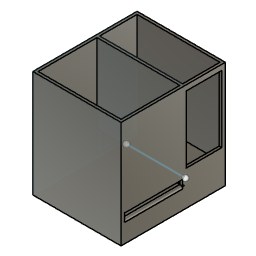
PVP v6 (Autodesk Fusion 360 design; units mm, degrees)
Autodesk Fusion 360 part; units mm, degrees
sketch "スケッチ1" plane through (0, 0, 0) normal (0, 0, 1) x (1, 0, 0)
  line L0 (-65, 35) -> (85, 35)
  line L1 (85, 35) -> (85, -65)
  line L2 (85, -65) -> (-65, -65)
  line L3 (-65, -65) -> (-65, 35)
  dimension "d1" = 150
  dimension "d2" = 100
  constraint horizontal L0
  constraint vertical L1
  constraint horizontal L2
  constraint vertical L3
  measures "d1" distance of L0.start L0.end
  measures "d2" distance of L0.start L2.end
extrude "押し出し1" add sketch "スケッチ1" along normal blind 10 makes body 1
move_body "移動1" bodies 1 to x (1, 0, 0) y (0, 1, 0) z (0, 0, 1) at (-187.9301, -38.7882, -61.9373)
sketch "スケッチ2" plane through (0, 0, 0) normal (0, 1, 0) x (1, 0, 0)
sketch "スケッチ3" plane through (0, 0, 0) normal (0, 0, 1) x (1, 0, 0)
  line L0 (-50, 110) -> (115, 110)
  line L1 (115, 110) -> (115, -85)
  line L2 (115, -85) -> (-50, -85)
  line L3 (-50, -85) -> (-50, 110)
  line L4 (-45, 105) -> (110, 105)
  line L5 (110, 105) -> (110, 35)
  line L6 (110, 35) -> (-45, 35)
  line L7 (-45, 35) -> (-45, 105)
  line L8 (-45, 30) -> (110, 30)
  line L9 (110, 30) -> (110, -80)
  line L10 (110, -80) -> (-45, -80)
  line L11 (-45, -80) -> (-45, 30)
  dimension "d5" = 165
  dimension "d6" = 195
  constraint horizontal L0
  constraint vertical L1
  constraint horizontal L2
  constraint vertical L3
  constraint horizontal L4
  constraint vertical L5
  constraint horizontal L6
  constraint vertical L7
  constraint horizontal L8
  constraint vertical L9
  constraint horizontal L10
  constraint vertical L11
  measures "d5" distance of L0.start L0.end
  measures "d6" distance of L0.start L2.end
extrude "押し出し2" add sketch "スケッチ3" along normal blind 200 separate body makes body 2
sketch "スケッチ4" plane through (0, 0, 0) normal (0, 0, 1) x (1, 0, 0)
  line L0 (-290, 140) -> (-125, 140)
  line L1 (-125, 140) -> (-125, -55)
  line L2 (-125, -55) -> (-290, -55)
  line L3 (-290, -55) -> (-290, 140)
  dimension "d9" = 165
  dimension "d10" = 195
  constraint horizontal L0
  constraint vertical L1
  constraint horizontal L2
  constraint vertical L3
  measures "d9" distance of L0.start L0.end
  measures "d10" distance of L0.start L2.end
extrude "押し出し3" add sketch "スケッチ4" along normal blind 5 separate body makes body 3
sketch "スケッチ5" plane through (115, 0, 0) normal (1, 0, 0) x (0, 1, 0)
  line L0 (-85, 0) -> (110, 0)
  line L1 (110, 0) -> (110, 200)
  line L2 (110, 200) -> (-85, 200)
  line L3 (-85, 200) -> (-85, 0)
  line L4 (37, 190) -> (103.5, 190)
  line L5 (103.5, 190) -> (103.5, 65)
  line L6 (103.5, 65) -> (37, 65)
  line L7 (37, 65) -> (37, 190)
  dimension "d13" = 66.5
  dimension "d14" = 125
  constraint horizontal L4
  constraint vertical L5
  constraint horizontal L6
  constraint vertical L7
  measures "d13" distance of L4.start L4.end
  measures "d14" distance of L4.start L6.end
extrude "押し出し4" cut sketch "スケッチ5" against normal blind 10 contours L4 L5 L6 L7 bodies 2
sketch "スケッチ6" plane through (-50, 0, 0) normal (-1, 0, 0) x (0, -1, 0)
  line L0 (-110, 0) -> (85, 0)
  line L1 (85, 0) -> (85, 200)
  line L2 (85, 200) -> (-110, 200)
  line L3 (-110, 200) -> (-110, 0)
  line L4 (-105, 40) -> (-40, 40)
  line L5 (-40, 40) -> (-40, 10)
  line L6 (-40, 10) -> (-105, 10)
  line L7 (-105, 10) -> (-105, 40)
  constraint horizontal L4
  constraint vertical L5
  constraint horizontal L6
  constraint vertical L7
extrude "押し出し5" cut sketch "スケッチ6" against normal blind 25 contours L4 L5 L6 L7 bodies 2
sketch "スケッチ7" plane through (0, 0, 0) normal (0, 0, 1) x (1, 0, 0)
  line L0 (110, 30) -> (-45, 30)
  line L1 (-45, 30) -> (-45, -80)
  line L2 (-45, -80) -> (110, -80)
  line L3 (110, -80) -> (110, 30)
  constraint horizontal L0
  constraint vertical L1
  constraint horizontal L2
  constraint vertical L3
move_body "移動2" bodies 2 to x (1, 0, 0) y (0, 1, 0) z (0, 0, 1) at (0, 0, -40)
extrude "押し出し6" add sketch "スケッチ7" against normal blind 5 bodies 2
move_face "面を移動1" by (0, 0, 45) 25 faces at (-45, -43.3333, 53.3333) (58.3333, -80, -16.6667) (6.6667, 30, -16.6667) (110, -6.6667, 53.3333) (-48.3333, 18.3333, -40) (60, -85, 26.6667) (6.6667, -6.6667, -5) (110, 59, -18.3333) (113.3333, 81.3333, 25) (5, 110, 26.6667) (6.6667, 30, 53.3333) (-45, 60, 106.6667) (-46.6667, 61.6667, -30) (58.3333, 35, 26.6667) (58.3333, -80, 53.3333) (6.6667, -6.6667, 0) (110, -6.6667, -16.6667) (-48.3333, 40, -10) (-48.3333, 18.3333, 160) (-50, 21.6667, 106.6667) (-46.6667, 83.3333, 0) (113.3333, 37, 66.6667) (113.3333, 103.5, 108.3333) (58.3333, 105, 40) (113.3333, 59.1667, 150) on bodies 2
sketch "スケッチ8" plane through (0, 30, 0) normal (0, -1, 0) x (1, 0, 0)
  line L0 (-45, 45) -> (110, 45)
  line L1 (110, 45) -> (110, 205)
  line L2 (110, 205) -> (-45, 205)
  line L3 (-45, 205) -> (-45, 45)
  line L4 (-45, 45) -> (110, 45)
  line L5 (110, 45) -> (110, 55)
  line L6 (110, 55) -> (-45, 55)
  line L7 (-45, 55) -> (-45, 45)
  constraint horizontal L4
  constraint vertical L5
  constraint horizontal L6
  constraint vertical L7
  constraint coincident L1 L5.end
  constraint coincident L0.start L3.end
extrude "押し出し7" cut sketch "スケッチ8" against normal blind 5 contours L0 L1 L3 L4 L5 L6 L7 bodies 2
sketch "スケッチ9" plane through (0, 35, 0) normal (0, 1, 0) x (-1, 0, 0)
  line L0 (-110, 55) -> (45, 55)
  line L1 (45, 55) -> (45, 205)
  line L2 (45, 205) -> (-110, 205)
  line L3 (-110, 205) -> (-110, 55)
  line L4 (-115, 55) -> (-5, 55)
  constraint perpendicular L3 L4
sketch "スケッチ10" plane through (115, 0, 0) normal (1, 0, 0) x (0, 1, 0)
  line L0 (103.5, 195) -> (103.5, 70)
  line L1 (103.5, 70) -> (37, 70)
  line L2 (37, 70) -> (37, 195)
  line L3 (37, 195) -> (103.5, 195)
  line L4 (-85, 5) -> (110, 5)
  line L5 (110, 5) -> (110, 205)
  line L6 (110, 205) -> (-85, 205)
  line L7 (-85, 205) -> (-85, 5)
  line L8 (-78.5, 55) -> (30.0664, 55)
  line L9 (30.0664, 55) -> (30.0664, 44.6907)
  line L10 (30.0664, 44.6907) -> (-78.5, 44.6907)
  line L11 (-78.5, 44.6907) -> (-78.5, 55)
  constraint horizontal L8
  constraint vertical L9
  constraint horizontal L10
  constraint vertical L11
extrude "押し出し8" cut sketch "スケッチ10" against normal blind 12 contours L8 L9 L10 L11 bodies 2
fillet "フィレット1" radius 10 1 edges at (110, -24.25, 55) on bodies 2
fillet "フィレット2" radius 5 1 edges at (115, -24.2168, 44.6907) on bodies 2
sketch "スケッチ11" plane through (0, 35, 0) normal (0, 1, 0) x (-1, 0, 0)
  line L0 (45, 45) -> (-110, 45)
  line L1 (-110, 45) -> (-110, 5)
  line L2 (-110, 5) -> (45, 5)
  line L3 (45, 5) -> (45, 45)
  line L4 (-110, 45) -> (-40, 45)
  line L5 (-40, 45) -> (-40, 40)
  line L6 (-40, 40) -> (-110, 40)
  line L7 (-110, 40) -> (-110, 45)
  dimension "d29" = 5
  constraint horizontal L4
  constraint vertical L5
  constraint horizontal L6
  constraint vertical L7
  constraint coincident L0.end L1.start
  measures "d29" distance of L0.end L6.end
extrude "押し出し9" add sketch "スケッチ11" along normal blind 70 contours L0 L1 L4 L5 L6 L7 bodies 2
sketch "スケッチ12" plane through (0, 0, 45) normal (0, 0, 1) x (-1, 0, 0)
  line L0 (-103, -30.0664) -> (-110, -30.0664)
  line L1 (-110, -30.0664) -> (-110, -105)
  line L2 (-110, -105) -> (-40, -105)
  line L3 (-40, -105) -> (-40, -35)
  line L4 (-40, -35) -> (45, -35)
  line L5 (45, -35) -> (45, 80)
  line L6 (45, 80) -> (-110, 80)
  line L7 (-110, 80) -> (-110, 78.5)
  line L8 (-110, 78.5) -> (-103, 78.5)
  line L9 (-103, 78.5) -> (-103, -30.0664)
  line L10 (-45, -35) -> (-68, -35)
  line L11 (-68, -35) -> (-68, -47.6)
  line L12 (-68, -47.6) -> (-45, -47.6)
  line L13 (-45, -47.6) -> (-45, -35)
  dimension "d32" = 23
  dimension "d33" = 12.6
  constraint horizontal L10
  constraint vertical L11
  constraint horizontal L12
  constraint vertical L13
  measures "d32" distance of L10.start L10.end
  measures "d33" distance of L10.start L12.end
extrude "押し出し10" cut sketch "スケッチ12" against normal blind 5 contours L10 L11 L12 L13 bodies 2
sketch "スケッチ13" plane through (0, 0, 40) normal (0, 0, -1) x (1, 0, 0)
  line L0 (68, -35) -> (68, -47.6)
  line L1 (68, -47.6) -> (45, -47.6)
  line L2 (45, -47.6) -> (45, -35)
  line L3 (45, -35) -> (40, -35)
  line L4 (40, -35) -> (40, -105)
  line L5 (40, -105) -> (110, -105)
  line L6 (110, -105) -> (110, -35)
  line L7 (110, -35) -> (68, -35)
  line L8 (68, -47.6) -> (73, -47.6)
  line L9 (73, -47.6) -> (73, -35)
  line L10 (73, -35) -> (68, -35)
  line L11 (68, -35) -> (68, -47.6)
  line L12 (45, -47.6) -> (40, -47.6)
  line L13 (40, -47.6) -> (40, -35)
  line L14 (40, -35) -> (45, -35)
  line L15 (45, -35) -> (45, -47.6)
  dimension "d36" = 5
  constraint horizontal L8
  constraint vertical L9
  constraint horizontal L10
  constraint vertical L11
  constraint coincident L7 L9.end
  constraint coincident L0.end L1.start
  constraint horizontal L12
  constraint vertical L13
  constraint horizontal L14
  constraint vertical L15
  constraint coincident L3.end L4.start
  constraint coincident L1.end L2.start
  measures "d36" distance of L0.end L8.end
extrude "押し出し11" add sketch "スケッチ13" along normal blind 35 contours L0 L7 L8 L9 L10 L11 | L2 L3 L4 L12 L13 L14 L15 bodies 2
sketch "スケッチ14" plane through (68, 0, 0) normal (-1, 0, 0) x (0, -1, 0)
  line L0 (-35, 45) -> (-47.6, 45)
  line L1 (-47.6, 45) -> (-47.6, 40)
  line L2 (-47.6, 40) -> (-47.6, 5)
  line L3 (-47.6, 5) -> (-35, 5)
  line L4 (-35, 5) -> (-35, 45)
  line L5 (-47.6, 34.1) -> (-35, 34.1)
  line L6 (-35, 34.1) -> (-35, 30)
  line L7 (-35, 30) -> (-47.6, 30)
  line L8 (-47.6, 30) -> (-47.6, 34.1)
  constraint horizontal L5
  constraint vertical L6
  constraint horizontal L7
  constraint vertical L8
  constraint coincident L4 L6.end
  constraint coincident L2 L5.start
extrude "押し出し12" add sketch "スケッチ14" along normal blind 4 contours L2 L4 L5 L6 L7 L8 bodies 2
sketch "スケッチ15" plane through (45, 0, 0) normal (1, 0, 0) x (0, 1, 0)
  line L0 (47.6, 45) -> (35, 45)
  line L1 (35, 45) -> (35, 5)
  line L2 (35, 5) -> (47.6, 5)
  line L3 (47.6, 5) -> (47.6, 40)
  line L4 (47.6, 40) -> (47.6, 45)
  line L5 (35, 34) -> (47.6, 34)
  line L6 (47.6, 34) -> (47.6, 29.9)
  line L7 (47.6, 29.9) -> (35, 29.9)
  line L8 (35, 29.9) -> (35, 34)
  dimension "d43" = 4.1
  constraint horizontal L5
  constraint vertical L6
  constraint horizontal L7
  constraint vertical L8
  constraint coincident L1 L5.start
  measures "d43" distance of L5.start L7.end
extrude "押し出し13" add sketch "スケッチ15" along normal blind 4 contours L1 L3 L5 L6 L7 L8 bodies 2
sketch "スケッチ16" plane through (-50, 0, 0) normal (-1, 0, 0) x (0, -1, 0)
  line L0 (-40, 45) -> (-40, 15)
  line L1 (-40, 15) -> (-105, 15)
  line L2 (-105, 15) -> (-105, 45)
  line L3 (-105, 45) -> (-40, 45)
  line L4 (-110, 5) -> (85, 5)
  line L5 (85, 5) -> (85, 205)
  line L6 (85, 205) -> (-110, 205)
  line L7 (-110, 205) -> (-110, 5)
sketch "スケッチ17" plane through (-50, 0, 0) normal (-1, 0, 0) x (0, -1, 0)
  line L0 (-40, 45) -> (-35, 45)
  line L1 (-35, 5) -> (-35, 45)
  line L2 (-35, 45) -> (-30, 45)
  constraint horizontal L0
  constraint perpendicular L0 L1
  constraint perpendicular L1 L2
sketch "スケッチ18" plane through (-50, 0, 0) normal (-1, 0, 0) x (0, -1, 0)
  line L0 (-33, 45) -> (-32, 45)
  line L1 (-32, 45) -> (-32, 42.5)
  line L2 (-32, 42.5) -> (-33, 42.5)
  line L3 (-33, 42.5) -> (-33, 45)
  line L4 (-33, 43.5) -> (-34, 43.5)
  line L5 (-34, 43.5) -> (-34, 42.5)
  line L6 (-34, 42.5) -> (-33, 42.5)
  line L7 (-33, 42.5) -> (-33, 43.5)
  line L8 (-32, 43.5) -> (-31, 43.5)
  line L9 (-31, 43.5) -> (-31, 42.5)
  line L10 (-31, 42.5) -> (-32, 42.5)
  line L11 (-32, 42.5) -> (-32, 43.5)
  constraint horizontal L0
  constraint vertical L1
  constraint horizontal L2
  constraint vertical L3
  constraint horizontal L4
  constraint vertical L5
  constraint horizontal L6
  constraint vertical L7
  constraint coincident L3 L4.start
  constraint horizontal L8
  constraint vertical L9
  constraint horizontal L10
  constraint vertical L11
  constraint coincident L1 L8.start
extrude "押し出し14" cut sketch "スケッチ18" against normal blind 164 bodies 2
sketch "スケッチ19" plane through (-50, 0, 0) normal (-1, 0, 0) x (0, -1, 0)
  line L0 (-33, 45) -> (-32, 45)
  line L1 (-32, 45) -> (-32, 47.5)
  line L2 (-32, 47.5) -> (-33, 47.5)
  line L3 (-33, 47.5) -> (-33, 45)
  constraint horizontal L0
  constraint vertical L1
  constraint horizontal L2
  constraint vertical L3
extrude "押し出し15" cut sketch "スケッチ19" against normal blind 10 bodies 2
sketch "スケッチ20" plane through (-50, 0, 0) normal (-1, 0, 0) x (0, -1, 0)
  line L0 (-132.5, 45) -> (-129.7, 45)
  line L1 (-129.7, 45) -> (-129.7, 44.1)
  line L2 (-129.7, 44.1) -> (-132.5, 44.1)
  line L3 (-132.5, 44.1) -> (-132.5, 45)
  line L4 (-131.1, 45) -> (-131.5, 45)
  line L5 (-131.5, 45) -> (-131.5, 48)
  line L6 (-131.5, 48) -> (-131.1, 48)
  line L7 (-131.1, 48) -> (-131.1, 45)
  line L8 (-131.1, 48) -> (-130.7, 48)
  line L9 (-130.7, 48) -> (-130.7, 45)
  line L10 (-130.7, 45) -> (-131.1, 45)
  line L11 (-131.1, 45) -> (-131.1, 48)
  dimension "d50" = 2.8
  dimension "d51" = 0.9
  dimension "d52" = 3
  constraint horizontal L0
  constraint vertical L1
  constraint horizontal L2
  constraint vertical L3
  constraint horizontal L4
  constraint vertical L5
  constraint horizontal L6
  constraint vertical L7
  constraint midpoint L0 L4.start
  constraint horizontal L8
  constraint vertical L9
  constraint horizontal L10
  constraint vertical L11
  constraint coincident L0 L9.end
  measures "d50" distance of L0.start L0.end
  measures "d51" distance of L0.start L2.end
  measures "d52" distance of L4.end L5.end
extrude "押し出し16" add sketch "スケッチ20" along normal blind 4 separate body makes body 4
move_body "移動3" bodies 4 to x (1, 0, 0) y (0, 1, 0) z (0, 0, 1) at (0, -98.6, -1.55)
hidden bodies 1 3
